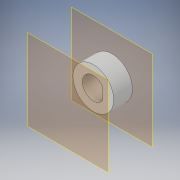
# Autodesk Inventor part: Hub Prototype
Saved by Autodesk Inventor 2018.2 (Build 222227000, 227)
## iProperties
Created: 2018-03-23
Part Number: Hub Prototype
Material: Generic
Document SubType Name: Modeling
Designer: MIABo
Density: 1 g/cm^3
Appearance: Default
Author: MIABo
## iProperties of the stored document Hub_3DPrint.ipt
Created: 2018-03-23
Part Number: Hub_3DPrint
Material: Generic
Document SubType Name: Modeling
Designer: MIABo
Density: 1 g/cm^3
Appearance: Default
Author: MIABo
Autodesk Inventor part; units mm, degrees
ref_plane "YZ Plane" through (0, 0, 0) normal (1, 0, 0) x (0, 1, 0)
ref_plane "XZ Plane" through (0, 0, 0) normal (0, 1, 0) x (-1, 0, 0)
ref_plane "XY Plane" through (0, 0, 0) normal (0, 0, 1) x (1, 0, 0)
ref_plane "Work Plane1" through (0, 0, 2.54) normal (0, 0, 1) x (1, 0, 0)
sketch "Sketch2" plane through (0, 0, 2.54) normal (0, 0, 1) x (1, 0, 0)
  circle A0 centre (0, 0) radius 5.5309
  dimension "d4" = 11.0617
  constraints: 1 centre point, 1 coincident
  measures "d4" diameter of A0
extrude "Extrusion2" add sketch "Sketch2" along normal blind 5.08
ref_plane "Work Plane2" through (0, 0, 14.5034) normal (0, 0, 1) x (1, 0, 0)
sketch "Sketch3" plane through (0, 0, 14.5034) normal (0, 0, 1) x (1, 0, 0)
  circle A0 centre (0, 0) radius 2.9909
  line L0 (2.5464, 1.5688) -> (2.5463, -1.5688)
  dimension "d7" = 5.9817
  dimension "d8" = 5.5372
  constraints: 2 end point, 2 point on circle, 1 centre point, 1 coincident, 1 vertical
  measures "d7" diameter of A0
extrude "Extrusion3" cut sketch "Sketch3" against normal blind 11.9634 contours L0 A0 picked at (1.7297, 0.9965)
body "Solid1"
